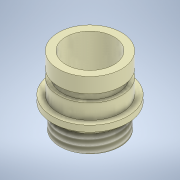
# Autodesk Inventor part: Conector Tapa-Corrugado V2
Saved by Autodesk Inventor 2020 (Build 240168000, 168)
## iProperties
Created: 2020-06-20
Part Number: Conector Tapa-Corrugado V2
Material: Polypropylene
Document SubType Name: Modeling
Designer: Juan
Density: 0.899 g/cm^3
Appearance: Smooth - Ash
Author: Juan
Autodesk Inventor part; units mm, degrees
ref_plane "YZ Plane" through (0, 0, 0) normal (1, 0, 0) x (0, 1, 0)
ref_plane "XZ Plane" through (0, 0, 0) normal (0, 1, 0) x (-1, 0, 0)
ref_plane "XY Plane" through (0, 0, 0) normal (0, 0, 1) x (1, 0, 0)
sketch "Sketch3" plane through (0, 0, 0) normal (0, 0, 1) x (1, 0, 0)
  line L0 (0, 0) -> (-10, 0)
  line L1 (-10, 0) -> (-10, 6)
  line L2 (-10, 6) -> (-10.25, 6)
  line L3 (-10.25, 6) -> (-10.25, 8)
  line L4 (-10.25, 8) -> (-12.5, 8)
  line L5 (-12.5, 8) -> (-12.5, 10)
  line L6 (-12.5, 10) -> (-10.5, 10)
  line L7 (-10.5, 10) -> (-10.5, 15)
  line L8 (-10.5, 15) -> (-9.2, 15)
  line L9 (-9.2, 15) -> (-9.2, 17.6)
  line L10 (-9.2, 17.6) -> (-10.5, 17.6)
  line L11 (-10.5, 17.6) -> (-10.5, 22.6)
  line L12 (-10.5, 22.6) -> (0, 22.6)
  line L13 (0, 22.6) -> (0, 0)
  line L14 (0, 22.6) -> (-8, 22.6)
  line L15 (-8, 22.6) -> (-8, 0)
  dimension "d23" = 10
  dimension "d24" = 6
  dimension "d25" = 0.25
  dimension "d26" = 2
  dimension "d27" = 2.25
  dimension "d28" = 2
  dimension "d29" = 2
  dimension "d30" = 5
  dimension "d31" = 1.3
  dimension "d32" = 2.6
  dimension "d33" = 5
  dimension "d34" = 8
  constraints: 32 end point, 11 perpendicular, 3 horizontal, 2 point on line, 1 vertical
  measures "d23" distance of L0.start L0.end
  measures "d24" distance of L0.end L1.end
  measures "d25" distance of L1.end L2.end
  measures "d26" distance of L2.end L3.end
  measures "d27" distance of L3.end L4.end
  measures "d28" distance of L4.end L5.end
  measures "d29" distance of L5.end L6.end
  measures "d30" distance of L6.end L7.end
  measures "d31" distance of L7.end L8.end
  measures "d32" distance of L8.end L9.end
  measures "d33" distance of L10.end L11.end
  measures "d34" distance of L12.end L14.end
revolve "Revolution2" add sketch "Sketch3" angle 360 about axis through (0, 22.6, 0) along (0, -1, 0) contours L0 L1 L2 L3 L4 L5 L6 L7 L8 L9 L10 L11 L12 L15
thread "Thread3" size "M20x2" class "6g" standard "ANSI Metric M Profile" full length
body "Solid2"
